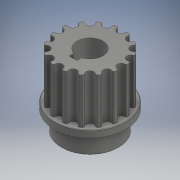
# Autodesk Inventor part: 15 tooth example pulley
Saved by Autodesk Inventor 2019.4 (Build 234330000, 330)
## iProperties
Created: 2017-06-13
Part Number: 15 tooth example pulley
Material: Steel
Document SubType Name: Modeling
Designer: Tobias
Density: 7.85 g/cm^3
Appearance: Anodized - Light Gray
Mass: 74.9849 g
Surface Area: 47.755 cm^2
Volume: 9.55222 cm^3
Author: Tobias
Autodesk Inventor part; units mm, degrees
ref_plane "YZ Plane" through (0, 0, 0) normal (1, 0, 0) x (0, 1, 0)
ref_plane "XZ Plane" through (0, 0, 0) normal (0, 1, 0) x (-1, 0, 0)
ref_plane "XY Plane" through (0, 0, 0) normal (0, 0, 1) x (1, 0, 0)
sketch "Sketch1" plane through (0, 0, 0) normal (0, 0, 1) x (1, 0, 0)
  circle A0 centre (0, 0) radius 12.73
  dimension "d0" = 25.46
  constraints: 1 centre point, 1 coincident
  measures "d0" diameter of A0
extrude "Extrusion1" add sketch "Sketch1" along normal mid plane 17.6
sketch "Sketch3" plane through (0, 0, 0) normal (0, 0, 1) x (1, 0, 0)
  circle A0 centre (0, 0) radius 12.73 projected
  line L0 (0, 19.32) -> (0, -19.32) projected
  arc A1 (-1.54, 12.09) -> (1.54, 12.09) centre (0, 12.09) ccw
  line L1 (-1.54, 17.09) -> (1.54, 17.09)
  line L2 (1.54, 17.09) -> (1.54, 12.09)
  line L3 (-1.54, 12.09) -> (-1.54, 17.09)
  circle A2 centre (0, 0) radius 12.73 projected
  point P0 (0, 10.55)
  point P1 (0, 12.73)
  dimension "d50" = 1.54
  dimension "d51" = 2.18
  dimension "d52" = 5
  constraints: 6 end point, 3 point on circle, 2 point on line, 2 tangent, 1 centre point, 1 horizontal, 1 parallel, 1 perpendicular, 1 vertical alignment, 1 other
  measures "d50" radius of A1
  measures "d51" distance of point (0, 10.55) point (0, 12.73)
  measures "d52" distance from line of A1.centre L1
extrude "Extrusion3" cut sketch "Sketch3" along normal mid plane 40 contours L2 A1 L0 A0 | A0 L0 L1 L2 | L0 A1 L3 A0 | A0 L3 L1 L0 picked at (0.3942, 12.0507) picked at (-0.3942, 12.0507)
pattern_circular "Circular Pattern2" count 16 over 360 about axis through (0, 0, -10) along (0, 0, 1) of "Extrusion3"
fillet "Fillet1" radius 0.5 2 edges at (-12.2639, -3.413, 0) (-12.6365, -1.54, 0)
pattern_circular "Circular Pattern3" count 16 over 360 about axis through (0, 0, -10) along (0, 0, 1) of "Fillet1"
sketch "Sketch5" plane through (0, 0, -8.8) normal (0, 0, -1) x (-1, 0, 0)
  circle A0 centre (0, 0) radius 13.8
  dimension "d24" = 27.6
  constraints: 1 centre point, 1 coincident
  measures "d24" diameter of A0
extrude "Extrusion5" add sketch "Sketch5" along normal blind 2.8
sketch "Sketch7" plane through (0, 0, -11.6) normal (0, 0, -1) x (-1, 0, 0)
  circle A0 centre (0, 0) radius 11.1
  dimension "d34" = 22.2
  constraints: 1 centre point, 1 coincident
  measures "d34" diameter of A0
extrude "Extrusion7" add sketch "Sketch7" along normal blind 7.4
sketch "Sketch8" plane through (0, 0, -19) normal (0, 0, -1) x (-1, 0, 0)
  circle A0 centre (0, 0) radius 5
  dimension "d37" = 10
  constraints: 1 centre point, 1 coincident
  measures "d37" diameter of A0
extrude "Extrusion8" cut sketch "Sketch8" against normal up to next
fillet "Fillet3" radius 0.2 2 edges at (13.8, 0, -8.8) (13.8, 0, -11.6)
chamfer "Chamfer2" distance 0.3 angle 45 1 edges at (11.1, 0, -19)
sketch "Sketch9" plane through (0, 0, -19) normal (0, 0, -1) x (-1, 0, 0)
  line L0 (0, -19.32) -> (0, 19.32) projected
  line L1 (-19.32, 0) -> (19.32, 0) projected
  line L2 (1.5, -6.6) -> (-1.5, -6.6)
  line L3 (-1.5, -6.6) -> (-1.5, -3.7742)
  line L4 (-1.5, -3.7742) -> (1.5, -3.7742)
  line L5 (1.5, -3.7742) -> (1.5, -6.6)
  point P0 (0, 0)
  point P1 (0, 5)
  dimension "d45" = 3
  dimension "d46" = 11.6
  constraints: 8 end point, 2 parallel, 1 horizontal, 1 perpendicular, 1 point on line, 1 other
  measures "d45" distance between parallel lines of L3 L5
  measures "d46" distance from line of point (0, 5) L2
extrude "Extrusion9" cut sketch "Sketch9" against normal blind 39.25
body "Solid1"
